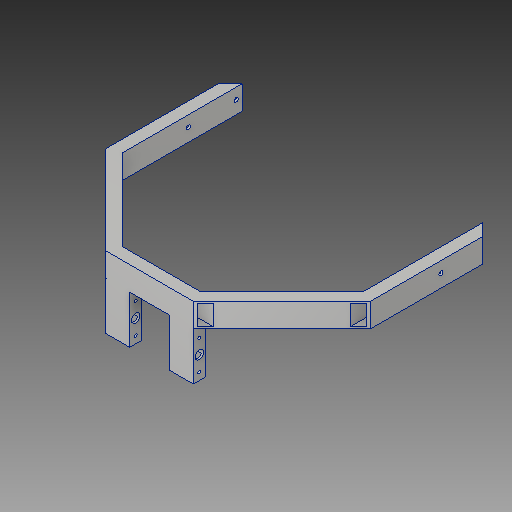
# Autodesk Inventor part: ShooterFrameV02
Saved by Autodesk Inventor 2017 SP1 (Build 210196100, 196)
## iProperties
Created: 2016-02-06
Part Number: ShooterFrameV02
Material: Aluminum 6061
Document SubType Name: Modeling
Designer: steele
Density: 2.7 g/cm^3
Appearance: Aluminum - Flat
Author: steele
Autodesk Inventor part; units mm, degrees
sketch "Sketch1" plane through (0, 0, 0) normal (0, 1, 0) x (-1, 0, 0)
  line L0 (0, 0) -> (201.6125, 0)
  line L1 (201.6125, 0) -> (201.6125, -330.2)
  line L2 (0, 0) -> (0, -330.2) construction
  line L3 (0, 0) -> (-201.6125, 0)
  line L4 (-201.6125, 0) -> (-201.6125, -330.2)
  dimension "d0" = 201.6125
  dimension "d1" = 330.2
  dimension "d2" = 330.2
  constraints: 10 end point, 2 symmetric about line, 1 horizontal, 1 perpendicular, 1 vertical
  measures "d0" distance of L0.start L0.end
  measures "d1" distance of L0.end L1.end
  measures "d2" distance of L0.start L2.end
ref_plane "Work Plane1" through (0, 0, -330.2) normal (0, 0, 1) x (1, 0, 0)
sketch "Sketch3" plane through (0, 0, -330.2) normal (0, 0, 1) x (1, 0, 0)
  line L0 (211.1375, -19.05) -> (192.0875, -19.05)
  line L1 (192.0875, -19.05) -> (192.0875, 19.05)
  line L2 (192.0875, 19.05) -> (211.1375, 19.05)
  line L3 (211.1375, 19.05) -> (211.1375, -19.05)
  line L4 (211.1375, -19.05) -> (192.0875, 19.05) construction
  line L5 (192.0875, -19.05) -> (211.1375, 19.05) construction
  line L6 (207.9625, -15.875) -> (195.2625, -15.875)
  line L7 (195.2625, -15.875) -> (195.2625, 15.875)
  line L8 (195.2625, 15.875) -> (207.9625, 15.875)
  line L9 (207.9625, 15.875) -> (207.9625, -15.875)
  line L10 (207.9625, -15.875) -> (195.2625, 15.875) construction
  line L11 (195.2625, -15.875) -> (207.9625, 15.875) construction
  point P0 (0, 0)
  point P1 (201.6125, 0)
  dimension "d4" = 38.1
  dimension "d5" = 19.05
  dimension "d6" = 201.6125
  dimension "d7" = 3.175
  dimension "d8" = 3.175
  constraints: 24 end point, 4 midpoint, 4 parallel, 2 horizontal, 2 perpendicular
  measures "d4" distance of L2.end L0.start
  measures "d5" distance of L0.start L0.end
  measures "d6" distance of point (201.612, 0) point (0, 0)
  measures "d7" distance between parallel lines of L2 L8
  measures "d8" distance between parallel lines of L3 L9
sweep "Sweep1" add profiles "Sketch3" path "Sketch1"
ref_plane "Work Plane2" through (-192.0875, -19.05, -9.525) normal (0, 0, 1) x (1, 0, 0)
sketch "Sketch12" plane through (-211.1375, 19.05, 9.525) normal (0, 1, 0) x (1, 0, 0)
  line L0 (406.4, 15.875) -> (15.875, 15.875) projected
  line L1 (19.05, 19.05) -> (19.05, 339.725) projected
  line L2 (19.05, 149.225) -> (149.225, 19.05)
  line L3 (403.225, 19.05) -> (19.05, 19.05) projected
  line L4 (19.05, 122.2842) -> (122.2842, 19.05)
  line L5 (19.05, 149.225) -> (19.05, 122.2842)
  line L6 (122.2842, 19.05) -> (149.225, 19.05)
  line L7 (211.1375, 9.525) -> (211.1375, 339.725) construction
  line L8 (403.225, 19.05) -> (403.225, 339.725)
  line L9 (403.225, 149.225) -> (273.05, 19.05)
  line L10 (19.05, 19.05) -> (403.225, 19.05)
  line L11 (403.225, 122.2842) -> (299.9908, 19.05)
  dimension "d50" = 130.175
  dimension "d51" = 130.175
  dimension "d52" = 19.05
  dimension "d55" = 330.2
  constraints: 18 end point, 8 point on line, 7 symmetric about line, 1 parallel, 1 vertical
  measures "d50" distance of L1.start L2.end
  measures "d51" distance of L2.start L1.start
  measures "d52" distance between parallel lines of L4 L2
  measures "d55" distance of L7.start L7.end
extrude "Extrusion5" add sketch "Sketch12" against normal blind 38.1 contours L9 L8 L11 L3 | L1 L2 L3 L4
sketch "Sketch14" plane through (-211.1375, 19.05, 9.525) normal (0, 1, 0) x (1, 0, 0)
  line L0 (0, 0) -> (0, 339.725) projected
  line L1 (0, 141.3342) -> (141.3342, 0)
  line L2 (422.275, 0) -> (0, 0) projected
  line L3 (19.05, 122.2842) -> (122.2842, 19.05) projected
  line L4 (0, 141.3342) -> (0, 0)
  line L5 (211.1375, 9.525) -> (211.1375, 339.725) construction
  dimension "d58" = 330.2
  constraints: 6 end point, 2 collinear, 2 point on line, 1 vertical
  measures "d58" distance of L5.start L5.end
extrude "Extrusion6" cut sketch "Sketch14" against normal blind 38.1
sketch "Sketch15" plane through (211.1375, 19.05, 9.525) normal (0, 1, 0) x (1, 0, 0)
  line L0 (0, 0) -> (-280.9408, 0) projected
  line L1 (-141.3342, 0) -> (0, 141.3342)
  line L2 (0, 339.725) -> (0, 0) projected
  line L3 (-122.2842, 19.05) -> (-19.05, 122.2842) projected
  line L4 (-141.3342, 0) -> (0, 0)
  point P0 (-211.1375, 9.525)
  constraints: 4 end point, 2 collinear, 2 point on line
extrude "Extrusion7" cut sketch "Sketch15" against normal blind 38.1
sketch "Sketch17" plane through (192.0875, 19.05, -330.2) normal (0, 1, 0) x (1, 0, 0)
  line L0 (-384.175, -190.5) -> (-384.175, 0) projected
  line L1 (-384.175, 0) -> (-403.225, -19.05)
  line L2 (-403.225, -198.3908) -> (-403.225, 0) projected
  line L3 (-403.225, -19.05) -> (-403.225, 0)
  line L4 (-403.225, 0) -> (-384.175, 0)
  point P0 (-192.0875, -330.2)
  dimension "d63" = 45
  constraints: 6 end point, 1 perpendicular, 1 point on line, 1 vertical
  measures "d63" angle of L0 L1
extrude "Extrusion8" cut sketch "Sketch17" against normal through all
sketch "Sketch18" plane through (192.0875, 19.05, -330.2) normal (0, 1, 0) x (1, 0, 0)
  line L0 (0, 0) -> (0, -190.5) projected
  line L1 (0, 0) -> (19.05, -19.05)
  line L2 (19.05, 0) -> (19.05, -198.3908) projected
  line L3 (19.05, -19.05) -> (19.05, 0)
  line L4 (19.05, 0) -> (0, 0) projected
  line L5 (19.05, 0) -> (0, 0)
  point P0 (-192.0875, -330.2)
  dimension "d66" = 45
  constraints: 6 end point, 2 collinear, 1 point on line
  measures "d66" angle of L1 L0
extrude "Extrusion9" cut sketch "Sketch18" against normal through all
sketch "Sketch19" plane through (-69.8033, -19.05, 9.525) normal (0, -1, 0) x (1, 0, 0)
  line L0 (139.6065, 0) -> (0, 0) projected
  line L1 (131.7158, -19.05) -> (7.8908, -19.05) projected
  line L2 (0, 0) -> (38.1, 0)
  line L3 (38.1, 0) -> (38.1, -19.05)
  line L4 (38.1, -19.05) -> (0, -19.05)
  line L5 (0, -19.05) -> (0, 0)
  line L6 (280.9408, -141.3342) -> (139.6065, 0) projected
  line L7 (139.6065, 0) -> (101.5065, 0)
  line L8 (101.5065, 0) -> (101.5065, -19.05)
  line L9 (101.5065, -19.05) -> (139.6065, -19.05)
  line L10 (139.6065, -19.05) -> (139.6065, 0)
  line L11 (0, -9.525) -> (139.6065, -9.525) construction
  line L12 (120.5565, 0) -> (120.5565, -19.05) construction
  line L13 (19.05, 0) -> (19.05, -19.05) construction
  line L14 (131.7158, -19.05) -> (7.8908, -19.05) construction
  line L15 (3.175, -15.875) -> (34.925, -15.875)
  line L16 (34.925, -15.875) -> (34.925, -3.175)
  line L17 (34.925, -3.175) -> (3.175, -3.175)
  line L18 (3.175, -3.175) -> (3.175, -15.875)
  line L19 (3.175, -15.875) -> (34.925, -3.175) construction
  line L20 (34.925, -15.875) -> (3.175, -3.175) construction
  line L21 (104.6815, -15.875) -> (136.4315, -15.875)
  line L22 (136.4315, -15.875) -> (136.4315, -3.175)
  line L23 (136.4315, -3.175) -> (104.6815, -3.175)
  line L24 (104.6815, -3.175) -> (104.6815, -15.875)
  line L25 (104.6815, -15.875) -> (136.4315, -3.175) construction
  line L26 (136.4315, -15.875) -> (104.6815, -3.175) construction
  point P0 (69.8033, -9.525)
  point P1 (19.05, -9.525)
  point P2 (120.5565, -9.525)
  dimension "d69" = 38.1
  dimension "d70" = 38.1
  dimension "d71" = 3.175
  dimension "d72" = 3.175
  dimension "d73" = 3.175
  dimension "d74" = 3.175
  constraints: 46 end point, 11 midpoint, 9 parallel, 4 perpendicular, 3 point on line, 2 horizontal
  measures "d69" distance between parallel lines of L3 L5
  measures "d70" distance between parallel lines of L8 L10
  measures "d71" distance between parallel lines of L3 L16
  measures "d72" distance between parallel lines of L17 L0
  measures "d73" distance between parallel lines of L23 L0
  measures "d74" distance between parallel lines of L8 L24
extrude "Extrusion10" add sketch "Sketch19" along normal blind 76.2 contours L10 L9 L1 L8 L0 | L3 L1 L4 L5 L0
sketch "Sketch20" plane through (69.8033, -19.05, 9.525) normal (1, 0, 0) x (0, 0, -1)
  circle A0 centre (9.525, -40.5384) radius 6.8707
  line L0 (141.3342, 0) -> (0, 0) projected
  point P0 (9.525, 19.05)
  dimension "d77" = 13.7414
  dimension "d78" = 40.5384
  constraints: 1 centre point
  measures "d77" diameter of A0
  measures "d78" distance from line of A0.centre L0
extrude "Extrusion11" cut sketch "Sketch20" against normal through all
ref_plane "Work Plane4" through (0, 19.05, -139.7) normal (-1, 0, 0) x (0, 0, -1)
ref_plane "Work Plane3" through (-192.0875, 19.05, -139.7) normal (-1, 0, 0) x (0, 0, -1)
sketch "Sketch21" plane through (-211.1375, -19.05, -131.8092) normal (-1, 0, 0) x (0, 0, 1)
  line L0 (-179.3408, 38.1) -> (-179.3408, 0) projected
  line L1 (0, 0) -> (-179.3408, 0) projected
  line L2 (0, 0) -> (0, 38.1) projected
  line L3 (0, 38.1) -> (-179.3408, 38.1) projected
  circle A0 centre (-112.6658, 20.6375) radius 3.3735 projected
  circle A1 centre (-188.8658, 20.6375) radius 3.3735 projected
  point P0 (131.8092, 19.05)
extrude "Extrusion12" cut sketch "Sketch21" against normal through all contours A0 | A1
sketch "Sketch22" plane through (69.8033, -19.05, 9.525) normal (1, 0, 0) x (0, 0, -1)
  circle A0 centre (9.525, -40.8462) radius 23.8125 construction
  arc A1 (15.875, -37.9147) -> (3.175, -37.9147) centre (9.525, -40.5384) ccw construction
  line L0 (9.525, -40.5384) -> (9.525, -17.0337) construction
  line L1 (9.525, -40.5384) -> (9.525, -64.6587) construction
  point P0 (9.525, 19.05)
  point P1 (-29.4266, 19.05)
  dimension "d84" = 47.625
  constraints: 4 end point, 2 coincident, 2 point on circle, 1 centre point, 1 point on line, 1 vertical
  measures "d84" diameter of A0
hole "Hole3" at (69.8033, 0, 38.9516) at (69.8033, -36.0837, 0) at (69.8033, -83.7087, 0) direction (-1, 0, 0) diameter 4.4958 end through all
equation "\"d0\" = 0.5 * width"
equation "\"d1\" = length"
equation "\"d2\" = length"
equation "\"d4\" = tubingLength"
equation "\"d5\" = tubingWidth"
equation "\"d6\" = 0.5 * width"
equation "\"d7\" = tubeingWallWidth"
equation "\"d8\" = tubeingWallWidth"
equation "\"d55\" = length"
equation "\"d58\" = length"
equation "\"d77\" = diamForAxel"
equation "\"width\" = 403.225"
equation "\"length\" = 330.2"
equation "\"tubingWidth\" = 19.05"
equation "\"tubingLength\" = 38.1"
equation "\"tubeingWallWidth\" = 3.175"
equation "\"d3\" = -length"
equation "\"diamForAxel\" = 13.7414"
body "Solid1"
